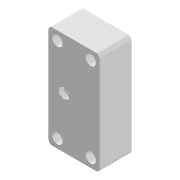
# Autodesk Inventor part: 10_Mountinplate_Mirrors_v0
Saved by Autodesk Inventor 2022.5 (Build 265521000, 521)
## iProperties
Created: 2022-05-18
Part Number: 10_Mountinplate_Mirrors_v0
Material: Generisch
Document SubType Name: Modeling
Designer: diederichbenedict
Density: 1 g/cm^3
Appearance: Vorgabe
Author: diederichbenedict
Autodesk Inventor part; units mm, degrees
ref_plane "Arbeitsebene1" through (7.9976, 1.0813, 0) normal (0, 0, 1) x (1, 0, 0)
sketch "Skizze1" plane through (7.9976, 1.0813, 0) normal (0, 0, 1) x (1, 0, 0)
  line L0 (0.635, 25.527) -> (10.16, 25.527) projected
  line L1 (0.635, 25.527) -> (0.635, 0) projected
  line L2 (0.635, 0) -> (10.16, 0) projected
  line L3 (10.16, 0) -> (10.16, 25.527) projected
  line L4 (30.08, -27.3) -> (-3.92, -27.3)
  line L5 (-6.92, -24.3) -> (-6.92, 49.7)
  line L6 (-3.92, 52.7) -> (30.08, 52.7)
  line L7 (33.08, -27.3) -> (-6.92, 52.7) construction
  line L8 (-6.92, -27.3) -> (33.08, 52.7) construction
  arc A0 (30.08, -27.3) -> (33.08, -24.3) centre (30.08, -24.3) ccw
  arc A1 (-6.92, -24.3) -> (-3.92, -27.3) centre (-3.92, -24.3) ccw
  arc A2 (-3.92, 52.7) -> (-6.92, 49.7) centre (-3.92, 49.7) ccw
  arc A3 (33.08, 49.7) -> (30.08, 52.7) centre (30.08, 49.7) ccw
  circle A4 centre (5.08, 12.7) radius 2.3813
  line L9 (33.08, -24.3) -> (33.08, 49.7)
  point P0 (-7.9976, -1.0813)
  point P1 (13.08, 12.7)
  dimension "d1" = 80
  dimension "d2" = 3
  dimension "d7" = 0
  dimension "d8" = 8
  constraints: 12 end point, 8 point on circle, 7 tangent, 6 point on line, 5 centre point, 3 equal radius, 1 horizontal, 1 midpoint, 1 parallel, 1 perpendicular, 1 vertical, 2 other
  measures "d1" distance of L8.start L7.end
  measures "d2" radius of A0
  measures "d7" vertical distance of A4.centre point (13.08, 12.7)
  measures "d8" distance of point (13.08, 12.7) A4.centre
ref_plane "Arbeitsebene2" through (291.5074, -13.3966, 8.6065) normal (0, 0, 1) x (0.898794, -0.4383711, 0)
extrude "Extrusion1" add sketch "Skizze1" along normal blind 23.612 contours L0 L3 L2 L1 | L4 A1 L5 A2 L6 A3 L9 A0
sketch "Skizze3" plane through (7.9976, 1.0813, 0) normal (0, 0, -1) x (-1, 0, 0)
  arc A0 (-30.08, 52.7) -> (-33.08, 49.7) centre (-30.08, 49.7) ccw projected
  line L0 (-33.08, -24.3) -> (-33.08, 49.7) projected
  arc A1 (-33.08, -24.3) -> (-30.08, -27.3) centre (-30.08, -24.3) ccw projected
  line L1 (3.92, -27.3) -> (-30.08, -27.3) projected
  arc A2 (3.92, -27.3) -> (6.92, -24.3) centre (3.92, -24.3) ccw projected
  line L2 (6.92, 49.7) -> (6.92, -24.3) projected
  arc A3 (6.92, 49.7) -> (3.92, 52.7) centre (3.92, 49.7) ccw projected
  line L3 (-30.08, 52.7) -> (3.92, 52.7) projected
  circle A4 centre (-5.08, 12.7) radius 2.3813 projected
  line L4 (-26.08, 45.7) -> (-0.08, 45.7)
  line L5 (-0.08, 45.7) -> (-0.08, -20.3)
  line L6 (-0.08, -20.3) -> (-26.08, -20.3)
  line L7 (-26.08, -20.3) -> (-26.08, 45.7)
  point P0 (7.9976, -1.0813)
  dimension "d9" = 7
  constraints: 8 end point, 3 other
  measures "d9" distance between parallel lines of L0 L7
hole "Bohrung1" at (34.0776, 46.7813, 0) at (34.0776, -19.2187, 0) at (8.0776, -19.2187, 0) at (8.0776, 46.7813, 0) direction (0, 0, 1) diameter 8 end through all
sketch "Skizze4" plane through (1.0776, -23.2187, 0) normal (-1, 0, 0) x (0, 0, 1)
  circle A0 centre (-6.731, 16.592) radius 9.366
  circle A1 centre (-6.731, 56.05) radius 7.366
  circle A2 centre (-6.731, 56.05) radius 9.366
  circle A3 centre (-6.7255, 16.9301) radius 7.366 projected
  point P0 (0, 23.2187)
  constraints: 3 centre point, 1 equal radius, 2 other
ref_plane "Arbeitsebene3" through (0, -11.176, -49.276) normal (-1, 0, 0) x (0, 0.0000004, 1)
extrude "Extrusion2" cut sketch "Skizze4" along normal up to surface (1.0776 mm away) contours A0 | A1 | A2 | A3
sketch "Skizze5" plane through (7.9976, 1.0813, 0) normal (0, 0, -1) x (-1, 0, 0)
  circle A0 centre (-5.08, 12.7) radius 2.3813 projected
  arc A1 (6.92, 49.7) -> (3.92, 52.7) centre (3.92, 49.7) ccw projected
  line L0 (-30.08, 52.7) -> (3.92, 52.7) projected
  arc A2 (-30.08, 52.7) -> (-33.08, 49.7) centre (-30.08, 49.7) ccw projected
  line L1 (-33.08, -24.3) -> (-33.08, 49.7) projected
  arc A3 (-33.08, -24.3) -> (-30.08, -27.3) centre (-30.08, -24.3) ccw projected
  line L2 (3.92, -27.3) -> (-30.08, -27.3) projected
  arc A4 (3.92, -27.3) -> (6.92, -24.3) centre (3.92, -24.3) ccw projected
  line L3 (6.92, 49.7) -> (6.92, -24.3) projected
  circle A5 centre (-0.08, 45.7) radius 4 projected
  circle A6 centre (-26.08, -20.3) radius 4 projected
  circle A7 centre (-26.08, 45.7) radius 4 projected
  circle A8 centre (-0.08, -20.3) radius 4 projected
  line L4 (3.7788, 28.1139) -> (-5.7462, 28.1139) projected
  line L5 (3.7788, -3.3013) -> (-5.7462, -3.3013) projected
  line L6 (-5.7462, -3.3013) -> (-5.7462, 28.1139)
  line L7 (3.7788, 28.1139) -> (3.7788, -3.3013)
  line L8 (0.0075, 0.2051) -> (0.0075, -12.8204) projected
  line L9 (-5.9462, 28.3139) -> (3.9788, 28.3139)
  line L10 (3.9788, 28.3139) -> (3.9788, -3.5013)
  line L11 (3.9788, -3.5013) -> (-5.9462, -3.5013)
  line L12 (-5.9462, -3.5013) -> (-5.9462, 28.3139)
  line L13 (-12.6873, 36.83) -> (-19.1643, 36.83)
  line L14 (-12.6873, -11.811) -> (-19.1643, -11.811)
  line L15 (-12.6873, 17.399) -> (-12.6873, 4.5974)
  line L16 (-19.7993, 21.1275) -> (-19.7993, 26.543)
  line L17 (-12.6873, -11.811) -> (-19.7993, -11.811)
  line L18 (-19.7993, -11.811) -> (-19.7993, 36.83)
  line L19 (-19.7993, 36.83) -> (-12.6873, 36.83)
  line L20 (-12.6873, 36.83) -> (-12.6873, -11.811)
  line L21 (-19.9993, 37.03) -> (-19.9993, -12.011)
  line L22 (-19.9993, -12.011) -> (-12.4873, -12.011)
  line L23 (-12.4873, -12.011) -> (-12.4873, 37.03)
  line L24 (-12.4873, 37.03) -> (-19.9993, 37.03)
  line L25 (-19.9993, -12.011) -> (-22.9993, -12.011)
  line L26 (-22.9993, -12.011) -> (-22.9993, 37.03)
  line L27 (-22.9993, 37.03) -> (-19.9993, 37.03)
  line L28 (-19.9993, 37.03) -> (-19.9993, -12.011)
  line L29 (0, -0.127) -> (0, 25.4)
  line L30 (0, -0.127) -> (0, 25.4)
  line L31 (3.9788, -3.5013) -> (0.0075, -3.5013)
  line L32 (0.2725, 0.2051) -> (0.2725, 25.2373)
  line L33 (4.6788, 26.5841) -> (3.9788, 26.5841)
  line L34 (3.9788, 26.5841) -> (3.9788, -3.5013)
  point P0 (7.9976, -1.0813)
  point P1 (0.0075, -12.8204)
  point P2 (0.0075, 0.2051)
  point P3 (-19.9993, 37.03)
  point P4 (7.5138, 27.9758)
  point P5 (3.9788, 26.5841)
  point P6 (7.5138, 27.9758)
  dimension "d20" = 0.2
  dimension "d26" = 0.2
  dimension "d27" = 3
  dimension "d28" = 0.7
  constraints: 56 end point, 8 parallel, 6 vertical, 5 horizontal, 4 perpendicular, 18 other
  measures "d20" distance between parallel lines of L7 L10
  measures "d26" distance between parallel lines of L18 L21
  measures "d27" distance of L26.end L27.end
  measures "d28" distance of L33.end L33.start
ref_plane "Arbeitsebene4" through (-0.1034, 27.5049, -1.27) normal (0, 0.0000004, 1) x (1, 0, 0)
extrude "Extrusion3" add sketch "Skizze5" along normal up to surface (1.27 mm away) contours A0 L6 | A0 L6 L4 L7 L5 | L6 A0 L12 | A0 L12 L9 L10 L11 L8 L5 L7 L4 L6 | L6 L5 L8 L11 L12 A0 | L12 A0 | L3 A4 L2 A3 L1 A2 L0 A1
sketch "Sketch6" plane through (7.9976, 1.0813, 23.612) normal (0, 0, 1) x (1, 0, 0)
  circle A0 centre (5.08, 12.7) radius 2.3813 projected
  line L0 (8.8085, 14.7861) -> (8.7509, 10.5141)
  line L1 (8.7509, 10.5141) -> (5.0224, 8.428)
  line L2 (5.0224, 8.428) -> (1.3515, 10.6139)
  line L3 (1.3515, 10.6139) -> (1.4091, 14.8859)
  line L4 (1.4091, 14.8859) -> (5.1376, 16.972)
  line L5 (5.1376, 16.972) -> (8.8085, 14.7861)
  point P0 (-7.9976, -1.0813)
  dimension "d23" = 3.7
  constraints: 12 end point, 1 coincident, 13 other
  measures "d23" distance from line of L4 A0.centre
extrude "Extrusion4" cut sketch "Sketch6" against normal blind 4 contours A0 | L0 L1 L2 L3 L4 L5
fillet "Fillet1" radius 0.5 6 edges at (30.9969, 13.5907, -1.27) (20.4849, 13.5907, -1.27) (29.4969, 38.1112, -1.27) (24.2409, 38.1112, -1.27) (29.4969, -10.9297, -1.27) (24.2409, -10.9297, -1.27)
